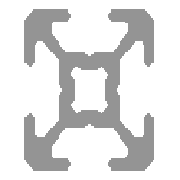
# Autodesk Inventor part: 2020x50mm
Saved by Autodesk Inventor 2015 (Build 190159000, 159)
## iProperties
Created: 2011-02-10
Part Number: 2020x50mm
Document SubType Name: Modeling
Designer: S. Wile
Density: 2.71 g/cm^3
Categories: <MemberInstance><Categories><Category DisplayName="Structural Shapes" InternalName="089c4875-fa83-4c05-b084-43b9cc11f5ed" Mnemonic="GRDR"><CategoryParameter DisplayName="Custom Base Point" InternalName="4f1d1b73-316d-484b-a3df-9cbabb16eb77" Mnemonic="shpBasePoint"/><CategoryParameter DisplayName="FG Authored" InternalName="9c666724-f362-4ea7-ac62-f6a007de5c69" Mnemonic="shpFGAuto"/><CategoryParameter DisplayName="Legacy Member ID" InternalName="340afe4f-75d7-48d3-ab7d-943f3c3da468" Mnemonic="LegacyMemberID"/><CategoryParameter DisplayName="Base Length" InternalName="42e34263-8f20-4d0e-ad48-bf1385b87c24" Mnemonic="shplen"/><CategoryParameter DisplayName="Distance of the Center of Gravity X-X" InternalName="26c9bdb8-9c79-4b4f-a92e-8e197583c9c4" Mnemonic="grcendistX"/><CategoryParameter DisplayName="Distance of the Center of Gravity Y-Y" InternalName="bcc4fb17-7af4-436a-8f8c-d0aa3b0248c5" Mnemonic="grcendistY"/><CategoryParameter DisplayName="Torsional Rigidity Modulus" InternalName="26c1ec35-5026-4c63-ad0a-751cf684a536" Mnemonic="torrigmod"/><CategoryParameter DisplayName="Torsional Section Modulus" InternalName="7c55a8dc-8844-49f9-a867-cc677b30ec9a" Mnemonic="torsecmod"/><CategoryParameter DisplayName="Coefficient of Shear Displacement" InternalName="de4c90c6-aaa8-468f-a335-6737b311b5d3" Mnemonic="shdispc"/><CategoryParameter DisplayName="Section Area" InternalName="1ff91680-64b0-4202-b9a3-7fd3f94bba3b" Mnemonic="secarea"/><CategoryParameter DisplayName="Moment of Inertia (x)" InternalName="4cd780bc-73d7-43ac-917a-579e5cbd684d" Mnemonic="inermomx"/><CategoryParameter DisplayName="Moment of Inertia (y)" InternalName="4b9f58ea-bced-460e-81ea-3d29ca5a49e3" Mnemonic="inermomy"/><CategoryParameter DisplayName="Section Module (x)" InternalName="72cfad18-cf51-4ed4-aaa7-c6b224f8419f" Mnemonic="secmodx"/><CategoryParameter DisplayName="Section Module (y)" InternalName="59eaa5e9-d227-48dc-b6c1-6920f96e0f95" Mnemonic="secmody"/><CategoryParameter DisplayName="Radius of Gyration (x)" InternalName="25778675-03e9-40c1-b6a8-4a9ed693320d" Mnemonic="gyrradx"/><CategoryParameter DisplayName="Radius of Gyration (y)" InternalName="bfa18ebe-1636-4dbe-8d42-b263e0b73184" Mnemonic="gyrrady"/><CategoryParameter DisplayName="Shape Thickness" InternalName="d109cf76-8eb4-42fc-9800-4409734adc67" Mnemonic="shpthick"/><CategoryParameter DisplayName="Second Shape Thickness" InternalName="9251a8e1-85fd-4e47-af99-afdb762317d9" Mnemonic="shpthick2"/><CategoryParameter DisplayName="Shape Width" InternalName="7c717d54-a18f-4666-b4d4-573cce22c62c" Mnemonic="shpwdth"/><CategoryParameter DisplayName="Shape Height" InternalName="50274e7d-5ac0-4796-92cb-c59e54983c67" Mnemonic="shpheig"/><CategoryParameter DisplayName="Mass per Length Unit" InternalName="0bb95a10-148f-4027-a459-38d7b056702a" Mnemonic="shpmass"/><CategoryParameter DisplayName="Section Designation" InternalName="5a64d034-428d-49c8-ba32-7619764de20f" Mnemonic="shpdes"/><Category DisplayName="Other" InternalName="f02205ff-2390-476f-921c-0b3185f88e84" Mnemonic="OTHSHP"><CategoryParameter DisplayName="Moment of Inertia (x)" InternalName="ec6737bc-264f-43ed-b0bd-f6d410c2718d" Mnemonic="inermomx"/><CategoryParameter DisplayName="Moment of Inertia (y)" InternalName="044c654e-f649-48ac-84cc-650a29ae31ca" Mnemonic="inermomy"/><CategoryParameter DisplayName="Section Module (x)" InternalName="cac70804-9d39-43bb-be17-56ea1f39a6c2" Mnemonic="secmodx"/><CategoryParameter DisplayName="Section Module (y)" InternalName="88b8bff9-a616-4028-93d5-ed4f79680d13" Mnemonic="secmody"/><CategoryParameter DisplayName="Section Area" InternalName="c46ecdf8-b6eb-4db9-8b25-30258930c1e3" Mnemonic="secarea"/><CategoryParameter DisplayName="Radius of Gyration (x)" InternalName="ee72c61e-565e-4fd6-b448-66e1e1abcb7e" Mnemonic="gyrradx"/><CategoryParameter DisplayName="Radius of Gyration (y)" InternalName="743e1dfe-1bba-408b-b985-cf752b207386" Mnemonic="gyrrady"/><CategoryParameter DisplayName="Shape Thickness" InternalName="12b1a788-9233-48fd-a933-2df8ff42b15f" Mnemonic="shpthick"/><CategoryParameter DisplayName="Mass per Length Unit" InternalName="2fd289d6-9394-4d2d-97e6-6659d7d4551d" Mnemonic="shpmass"/></Category></Category></Categories><FamilyTemplate Id="20x20"><FamilyTemplateParameters><FamilyTemplateParameter ObjectType="kUserParameterObject" ValueType="xs:double" Id="1" ObjectReferenceKey="Length"/><FamilyTemplateParameter ObjectType="kPropertyObject" ValueType="xs:string" Id="4" ObjectReferenceKey="{32853F0F-3444-11d1-9E93-0060B03C1CA6}" SubObjectId="52"/><FamilyTemplateParameter ObjectType="kPartComponentDefinitionObject" ValueType="xs:string" Id="5" SubObjectId="Material"/><FamilyTemplateParameter ObjectType="kPropertyObject" ValueType="xs:string" Id="6" ObjectReferenceKey="{32853F0F-3444-11d1-9E93-0060B03C1CA6}" SubObjectId="5"/><FamilyTemplateParameter ObjectType="kPropertyObject" ValueType="xs:string" Id="7" ObjectReferenceKey="{32853F0F-3444-11D1-9E93-0060B03C1CA6}" SubObjectId="55"/><FamilyTemplateParameter ObjectType="kiPartTableColumnObject" ValueType="xs:string" Id="18" ObjectReferenceKey="FILENAME"/><FamilyTemplateParameter ObjectType="kiPartTableColumnObject" ValueType="xs:string" Id="19" ObjectReferenceKey="MEMBER_REVISION"/></FamilyTemplateParameters></FamilyTemplate><CategoryParameterMap><ParamToTemplateMap><ParamToTemplate CategoryParameter="//CategoryParameter[@InternalName='9c666724-f362-4ea7-ac62-f6a007de5c69']" ConstantValue="1"/><ParamToTemplate CategoryParameter="//CategoryParameter[@InternalName='2675968c-4ce5-49e0-a4f5-552d29089031']" TemplateParameter="4"/><ParamToTemplate CategoryParameter="//CategoryParameter[@InternalName='8b46a4cc-9585-4fed-90c3-899f57e09a73']" TemplateParameter="18"/><ParamToTemplate CategoryParameter="//CategoryParameter[@InternalName='42e34263-8f20-4d0e-ad48-bf1385b87c24']" TemplateParameter="1"/><ParamToTemplate CategoryParameter="//CategoryParameter[@InternalName='818a152a-d3c3-49ca-80ee-df7d91421b8e']" TemplateParameter="5"/><ParamToTemplate CategoryParameter="//CategoryParameter[@InternalName='a65d44b9-392f-4f4f-857b-e4b3d54996fe']" TemplateParameter="19"/><ParamToTemplate CategoryParameter="//CategoryParameter[@InternalName='016b6077-bfbe-49bd-92c9-d8d59c39c941']" TemplateParameter="6"/></ParamToTemplateMap></CategoryParameterMap></MemberInstance>
Stock Number: 3 842 992 888
Description: PROFILE 20x20, -/-
Material: Aluminum-6061
Mass: 11.2397 g
Surface Area: 47.9691 cm^2
Volume: 4.14751 cm^3
Appearance: Aluminum - Flat-1
RuleStatus: InUse
Author: S. Wile
Autodesk Inventor part; units mm, degrees
ref_plane "YZ Plane" through (0, 0, 0) normal (1, 0, 0) x (0, 1, 0)
ref_plane "XZ Plane" through (0, 0, 0) normal (0, 1, 0) x (-1, 0, 0)
ref_plane "XY Plane" through (0, 0, 0) normal (0, 0, 1) x (1, 0, 0)
sketch "20x20" plane through (0, 0, 0) normal (0, 0, 1) x (1, 0, 0)
  line L0 (-14.2327, 14.1046) -> (-14.2327, 14.8364)
  arc A0 (-14.2327, 14.1046) -> (-13.7327, 13.6046) centre (-13.7327, 14.1046) ccw
  line L1 (-11.7327, 13.6046) -> (-13.7327, 13.6046)
  arc A1 (-11.2327, 13.1046) -> (-11.7327, 13.6046) centre (-11.7327, 13.1046) ccw
  line L2 (-11.2327, 12.8046) -> (-11.2327, 13.1046)
  arc A2 (-11.4327, 12.6046) -> (-11.2327, 12.8046) centre (-11.4327, 12.8046) ccw
  line L3 (-11.5818, 12.6046) -> (-11.4327, 12.6046)
  arc A3 (-11.5818, 12.6046) -> (-11.7818, 12.4046) centre (-11.5818, 12.4046) ccw
  line L4 (-11.7818, 12.3042) -> (-11.7818, 12.4046)
  arc A4 (-11.9818, 12.1042) -> (-11.7818, 12.3042) centre (-11.9818, 12.3042) ccw
  line L5 (-16.7331, 12.1042) -> (-11.9818, 12.1042)
  arc A5 (-18.2331, 13.6042) -> (-16.7331, 12.1042) centre (-16.7331, 13.6042) ccw
  line L6 (-18.2331, 18.3542) -> (-18.2331, 13.6042)
  arc A6 (-18.0331, 18.5542) -> (-18.2331, 18.3542) centre (-18.0331, 18.3542) ccw
  line L7 (-17.9323, 18.5542) -> (-18.0331, 18.5542)
  arc A7 (-17.9323, 18.5542) -> (-17.7323, 18.7542) centre (-17.9323, 18.7542) ccw
  line L8 (-17.7323, 18.9046) -> (-17.7323, 18.7542)
  arc A8 (-17.5323, 19.1046) -> (-17.7323, 18.9046) centre (-17.5323, 18.9046) ccw
  line L9 (-17.2323, 19.1046) -> (-17.5323, 19.1046)
  arc A9 (-16.7323, 18.6046) -> (-17.2323, 19.1046) centre (-17.2323, 18.6046) ccw
  line L10 (-16.7323, 16.6045) -> (-16.7323, 18.6046)
  arc A10 (-16.7323, 16.6045) -> (-16.2323, 16.1045) centre (-16.2323, 16.6045) ccw
  line L11 (-15.5001, 16.1045) -> (-16.2323, 16.1045)
  arc A11 (-15.5001, 16.1045) -> (-15.1465, 16.251) centre (-15.5001, 16.6045) ccw
  line L12 (-12.8787, 18.5188) -> (-15.1465, 16.251)
  arc A12 (-12.8787, 18.5188) -> (-12.7323, 18.8723) centre (-13.2323, 18.8723) ccw
  line L13 (-12.7323, 21.1509) -> (-12.7323, 18.8723)
  arc A13 (-12.7055, 21.2509) -> (-12.7323, 21.1509) centre (-12.5323, 21.1509) ccw
  line L14 (-12.2704, 22.0045) -> (-12.7055, 21.2509)
  arc A14 (-12.2704, 22.0045) -> (-12.2704, 22.2045) centre (-12.4436, 22.1045) ccw
  line L15 (-12.7055, 22.9581) -> (-12.2704, 22.2045)
  arc A15 (-12.7323, 23.0581) -> (-12.7055, 22.9581) centre (-12.5323, 23.0581) ccw
  line L16 (-12.7323, 25.3364) -> (-12.7323, 23.0581)
  arc A16 (-12.7323, 25.3364) -> (-12.8787, 25.69) centre (-13.2323, 25.3364) ccw
  line L17 (-15.1465, 27.9577) -> (-12.8787, 25.69)
  arc A17 (-15.1465, 27.9577) -> (-15.5001, 28.1042) centre (-15.5001, 27.6042) ccw
  line L18 (-16.2323, 28.1042) -> (-15.5001, 28.1042)
  arc A18 (-16.2323, 28.1042) -> (-16.7323, 27.6042) centre (-16.2323, 27.6042) ccw
  line L19 (-16.7323, 25.6038) -> (-16.7323, 27.6042)
  arc A19 (-17.2323, 25.1038) -> (-16.7323, 25.6038) centre (-17.2323, 25.6038) ccw
  line L20 (-17.5323, 25.1038) -> (-17.2323, 25.1038)
  arc A20 (-17.7323, 25.3038) -> (-17.5323, 25.1038) centre (-17.5323, 25.3038) ccw
  line L21 (-17.7323, 25.452) -> (-17.7323, 25.3038)
  arc A21 (-17.7323, 25.452) -> (-17.9323, 25.652) centre (-17.9323, 25.452) ccw
  line L22 (-18.0331, 25.652) -> (-17.9323, 25.652)
  arc A22 (-18.2331, 25.852) -> (-18.0331, 25.652) centre (-18.0331, 25.852) ccw
  line L23 (-18.2331, 30.602) -> (-18.2331, 25.852)
  arc A23 (-16.7331, 32.102) -> (-18.2331, 30.602) centre (-16.7331, 30.602) ccw
  arc A24 (-11.7818, 31.8042) -> (-11.5818, 31.6042) centre (-11.5818, 31.8042) ccw
  line L24 (-11.4327, 31.6042) -> (-11.5818, 31.6042)
  arc A25 (-11.2327, 31.4042) -> (-11.4327, 31.6042) centre (-11.4327, 31.4042) ccw
  line L25 (-11.2327, 31.1042) -> (-11.2327, 31.4042)
  arc A26 (-11.7327, 30.6042) -> (-11.2327, 31.1042) centre (-11.7327, 31.1042) ccw
  line L26 (-13.7327, 30.6042) -> (-11.7327, 30.6042)
  arc A27 (-13.7327, 30.6042) -> (-14.2327, 30.1042) centre (-13.7327, 30.1042) ccw
  line L27 (-14.2327, 29.3723) -> (-14.2327, 30.1042)
  arc A28 (-14.2327, 29.3723) -> (-14.0862, 29.0188) centre (-13.7327, 29.3723) ccw
  line L28 (-11.8181, 26.7506) -> (-14.0862, 29.0188)
  arc A29 (-11.8181, 26.7506) -> (-11.4646, 26.6042) centre (-11.4646, 27.1042) ccw
  line L29 (-9.1859, 26.6042) -> (-11.4646, 26.6042)
  arc A30 (-9.0859, 26.5774) -> (-9.1859, 26.6042) centre (-9.1859, 26.4042) ccw
  line L30 (-8.3323, 26.1423) -> (-9.0859, 26.5774)
  arc A31 (-8.3323, 26.1423) -> (-8.1323, 26.1423) centre (-8.2323, 26.3155) ccw
  line L31 (-7.3787, 26.5774) -> (-8.1323, 26.1423)
  arc A32 (-7.2787, 26.6042) -> (-7.3787, 26.5774) centre (-7.2787, 26.4042) ccw
  line L32 (-5.0004, 26.6042) -> (-7.2787, 26.6042)
  arc A33 (-5.0004, 26.6042) -> (-4.6469, 26.7506) centre (-5.0004, 27.1042) ccw
  line L33 (-2.3787, 29.0188) -> (-4.6469, 26.7506)
  arc A34 (-2.3787, 29.0188) -> (-2.2323, 29.3723) centre (-2.7323, 29.3723) ccw
  line L34 (-2.2323, 30.1042) -> (-2.2323, 29.3723)
  arc A35 (-2.2323, 30.1042) -> (-2.7323, 30.6042) centre (-2.7323, 30.1042) ccw
  line L35 (-4.7327, 30.6042) -> (-2.7323, 30.6042)
  arc A36 (-5.2327, 31.1042) -> (-4.7327, 30.6042) centre (-4.7327, 31.1042) ccw
  line L36 (-5.2327, 31.4042) -> (-5.2327, 31.1042)
  arc A37 (-5.0327, 31.6042) -> (-5.2327, 31.4042) centre (-5.0327, 31.4042) ccw
  line L37 (-4.884, 31.6042) -> (-5.0327, 31.6042)
  arc A38 (-4.884, 31.6042) -> (-4.684, 31.8042) centre (-4.884, 31.8042) ccw
  line L38 (-4.684, 31.902) -> (-4.684, 31.8042)
  arc A39 (-4.484, 32.102) -> (-4.684, 31.902) centre (-4.484, 31.902) ccw
  line L39 (0.2656, 32.102) -> (-4.484, 32.102)
  arc A40 (1.7656, 30.602) -> (0.2656, 32.102) centre (0.2656, 30.602) ccw
  line L40 (1.7656, 25.852) -> (1.7656, 30.602)
  arc A41 (1.5656, 25.652) -> (1.7656, 25.852) centre (1.5656, 25.852) ccw
  line L41 (1.467, 25.652) -> (1.5656, 25.652)
  arc A42 (1.467, 25.652) -> (1.267, 25.452) centre (1.467, 25.452) ccw
  line L42 (1.267, 25.3038) -> (1.267, 25.452)
  arc A43 (1.067, 25.1038) -> (1.267, 25.3038) centre (1.067, 25.3038) ccw
  line L43 (0.767, 25.1038) -> (1.067, 25.1038)
  arc A44 (0.267, 25.6038) -> (0.767, 25.1038) centre (0.767, 25.6038) ccw
  line L44 (0.267, 27.6042) -> (0.267, 25.6038)
  arc A45 (0.267, 27.6042) -> (-0.233, 28.1042) centre (-0.233, 27.6042) ccw
  line L45 (-0.965, 28.1042) -> (-0.233, 28.1042)
  arc A46 (-0.965, 28.1042) -> (-1.3185, 27.9577) centre (-0.965, 27.6042) ccw
  line L46 (-3.5862, 25.6901) -> (-1.3185, 27.9577)
  arc A47 (-3.5862, 25.6901) -> (-3.7326, 25.3365) centre (-3.2326, 25.3365) ccw
  line L47 (-3.7326, 23.0581) -> (-3.7326, 25.3365)
  arc A48 (-3.7594, 22.9581) -> (-3.7326, 23.0581) centre (-3.9326, 23.0581) ccw
  line L48 (-4.1945, 22.2045) -> (-3.7594, 22.9581)
  arc A49 (-4.1945, 22.2045) -> (-4.1945, 22.0045) centre (-4.0213, 22.1045) ccw
  line L49 (-3.7594, 21.2509) -> (-4.1945, 22.0045)
  arc A50 (-3.7326, 21.1509) -> (-3.7594, 21.2509) centre (-3.9326, 21.1509) ccw
  line L50 (-3.7326, 18.8723) -> (-3.7326, 21.1509)
  arc A51 (-3.7326, 18.8723) -> (-3.5862, 18.5187) centre (-3.2326, 18.8723) ccw
  line L51 (-1.3184, 16.251) -> (-3.5862, 18.5187)
  arc A52 (-1.3184, 16.251) -> (-0.9649, 16.1045) centre (-0.9649, 16.6045) ccw
  line L52 (-0.233, 16.1045) -> (-0.9649, 16.1045)
  arc A53 (-0.233, 16.1045) -> (0.267, 16.6045) centre (-0.233, 16.6045) ccw
  line L53 (0.267, 18.6046) -> (0.267, 16.6045)
  arc A54 (0.767, 19.1046) -> (0.267, 18.6046) centre (0.767, 18.6046) ccw
  line L54 (1.067, 19.1046) -> (0.767, 19.1046)
  arc A55 (1.267, 18.9046) -> (1.067, 19.1046) centre (1.067, 18.9046) ccw
  line L55 (1.267, 18.7542) -> (1.267, 18.9046)
  arc A56 (1.267, 18.7542) -> (1.467, 18.5542) centre (1.467, 18.7542) ccw
  line L56 (1.5656, 18.5542) -> (1.467, 18.5542)
  arc A57 (1.7656, 18.3542) -> (1.5656, 18.5542) centre (1.5656, 18.3542) ccw
  line L57 (1.7656, 13.6042) -> (1.7656, 18.3542)
  arc A58 (0.2656, 12.1042) -> (1.7656, 13.6042) centre (0.2656, 13.6042) ccw
  line L58 (-4.484, 12.1042) -> (0.2656, 12.1042)
  arc A59 (-4.684, 12.3042) -> (-4.484, 12.1042) centre (-4.484, 12.3042) ccw
  line L59 (-4.684, 12.4046) -> (-4.684, 12.3042)
  arc A60 (-4.684, 12.4046) -> (-4.884, 12.6046) centre (-4.884, 12.4046) ccw
  line L60 (-5.0327, 12.6046) -> (-4.884, 12.6046)
  arc A61 (-5.2327, 12.8046) -> (-5.0327, 12.6046) centre (-5.0327, 12.8046) ccw
  line L61 (-5.2327, 13.1046) -> (-5.2327, 12.8046)
  arc A62 (-4.7327, 13.6046) -> (-5.2327, 13.1046) centre (-4.7327, 13.1046) ccw
  line L62 (-2.7323, 13.6046) -> (-4.7327, 13.6046)
  arc A63 (-2.7323, 13.6046) -> (-2.2323, 14.1046) centre (-2.7323, 14.1046) ccw
  line L63 (-2.2323, 14.8364) -> (-2.2323, 14.1046)
  arc A64 (-2.2323, 14.8364) -> (-2.3788, 15.19) centre (-2.7323, 14.8364) ccw
  line L64 (-4.6465, 17.4577) -> (-2.3788, 15.19)
  arc A65 (-4.6465, 17.4577) -> (-5.0001, 17.6042) centre (-5.0001, 17.1042) ccw
  line L65 (-7.2787, 17.6042) -> (-5.0001, 17.6042)
  arc A66 (-7.3787, 17.631) -> (-7.2787, 17.6042) centre (-7.2787, 17.8042) ccw
  line L66 (-8.1323, 18.0661) -> (-7.3787, 17.631)
  arc A67 (-8.1323, 18.0661) -> (-8.3323, 18.0661) centre (-8.2323, 17.8929) ccw
  line L67 (-9.0859, 17.631) -> (-8.3323, 18.0661)
  arc A68 (-9.1859, 17.6042) -> (-9.0859, 17.631) centre (-9.1859, 17.8042) ccw
  line L68 (-11.4649, 17.6042) -> (-9.1859, 17.6042)
  arc A69 (-11.4649, 17.6042) -> (-11.8185, 17.4577) centre (-11.4649, 17.1042) ccw
  line L69 (-14.0862, 15.19) -> (-11.8185, 17.4577)
  arc A70 (-14.0862, 15.19) -> (-14.2327, 14.8364) centre (-13.7327, 14.8364) ccw
  line L70 (-11.2243, 24.0126) -> (-10.6774, 23.3609)
  arc A71 (-10.6774, 23.3609) -> (-10.6774, 20.8453) centre (-8.2329, 22.1031) ccw
  line L71 (-10.6774, 20.8453) -> (-11.2243, 20.1936)
  arc A72 (-11.2243, 20.1936) -> (-10.1463, 19.1142) centre (-8.2329, 22.1031) ccw
  line L72 (-10.1463, 19.1142) -> (-9.4907, 19.6586)
  arc A73 (-9.4907, 19.6586) -> (-6.9751, 19.6586) centre (-8.2329, 22.1031) ccw
  line L73 (-6.9751, 19.6586) -> (-6.3194, 19.1142)
  arc A74 (-6.3194, 19.1142) -> (-5.2414, 20.1936) centre (-8.2329, 22.1031) ccw
  line L74 (-5.2414, 20.1936) -> (-5.7884, 20.8453)
  arc A75 (-5.7884, 20.8453) -> (-5.7884, 23.3609) centre (-8.2329, 22.1031) ccw
  line L75 (-5.7884, 23.3609) -> (-5.2414, 24.0126)
  arc A76 (-5.2414, 24.0126) -> (-6.3195, 25.092) centre (-8.2329, 22.1031) ccw
  line L76 (-6.3195, 25.092) -> (-6.9751, 24.5476)
  arc A77 (-6.9751, 24.5476) -> (-9.4906, 24.5477) centre (-8.2329, 22.1031) ccw
  line L77 (-9.4906, 24.5477) -> (-10.1463, 25.092)
  arc A78 (-10.1463, 25.092) -> (-11.2243, 24.0126) centre (-8.2329, 22.1031) ccw
  line L78 (-11.9818, 32.102) -> (-16.7331, 32.102)
  arc A79 (-11.7818, 31.902) -> (-11.9818, 32.102) centre (-11.9818, 31.902) ccw
  line L79 (-11.7818, 31.8042) -> (-11.7818, 31.902)
sketch "Sketch1" plane through (0, 0, 0) normal (0, 0, 1) x (1, 0, 0)
  line L0 (-5.9998, -7.9985) -> (-5.9998, -7.2667)
  arc A0 (-5.9998, -7.9985) -> (-5.4998, -8.4985) centre (-5.4998, -7.9985) ccw
  line L1 (-3.4998, -8.4985) -> (-5.4998, -8.4985)
  arc A1 (-2.9998, -8.9985) -> (-3.4998, -8.4985) centre (-3.4998, -8.9985) ccw
  line L2 (-2.9998, -9.2985) -> (-2.9998, -8.9985)
  arc A2 (-3.1998, -9.4985) -> (-2.9998, -9.2985) centre (-3.1998, -9.2985) ccw
  line L3 (-3.3489, -9.4985) -> (-3.1998, -9.4985)
  arc A3 (-3.3489, -9.4985) -> (-3.5489, -9.6985) centre (-3.3489, -9.6985) ccw
  line L4 (-3.5489, -9.7989) -> (-3.5489, -9.6985)
  arc A4 (-3.7489, -9.9989) -> (-3.5489, -9.7989) centre (-3.7489, -9.7989) ccw
  line L5 (-8.5002, -9.9989) -> (-3.7489, -9.9989)
  arc A5 (-10.0002, -8.4989) -> (-8.5002, -9.9989) centre (-8.5002, -8.4989) ccw
  line L6 (-10.0002, -3.7489) -> (-10.0002, -8.4989)
  arc A6 (-9.8002, -3.5489) -> (-10.0002, -3.7489) centre (-9.8002, -3.7489) ccw
  line L7 (-9.6994, -3.5489) -> (-9.8002, -3.5489)
  arc A7 (-9.6994, -3.5489) -> (-9.4994, -3.3489) centre (-9.6994, -3.3489) ccw
  line L8 (-9.4994, -3.1985) -> (-9.4994, -3.3489)
  arc A8 (-9.2994, -2.9985) -> (-9.4994, -3.1985) centre (-9.2994, -3.1985) ccw
  line L9 (-8.9994, -2.9985) -> (-9.2994, -2.9985)
  arc A9 (-8.4994, -3.4985) -> (-8.9994, -2.9985) centre (-8.9994, -3.4985) ccw
  line L10 (-8.4994, -5.4986) -> (-8.4994, -3.4985)
  arc A10 (-8.4994, -5.4986) -> (-7.9994, -5.9986) centre (-7.9994, -5.4986) ccw
  line L11 (-7.2672, -5.9986) -> (-7.9994, -5.9986)
  arc A11 (-7.2672, -5.9986) -> (-6.9136, -5.8521) centre (-7.2672, -5.4986) ccw
  line L12 (-4.6458, -3.5844) -> (-6.9136, -5.8521)
  arc A12 (-4.6458, -3.5844) -> (-4.4994, -3.2308) centre (-4.9994, -3.2308) ccw
  line L13 (-4.4994, -0.9522) -> (-4.4994, -3.2308)
  arc A13 (-4.4726, -0.8522) -> (-4.4994, -0.9522) centre (-4.2994, -0.9522) ccw
  line L14 (-4.0375, -0.0986) -> (-4.4726, -0.8522)
  arc A14 (-4.0375, -0.0986) -> (-4.0375, 0.1014) centre (-4.2107, 0.0014) ccw
  line L15 (-4.4726, 0.855) -> (-4.0375, 0.1014)
  arc A15 (-4.4994, 0.955) -> (-4.4726, 0.855) centre (-4.2994, 0.955) ccw
  line L16 (-4.4994, 3.2333) -> (-4.4994, 0.955)
  arc A16 (-4.4994, 3.2333) -> (-4.6458, 3.5869) centre (-4.9994, 3.2333) ccw
  line L17 (-6.9136, 5.8546) -> (-4.6458, 3.5869)
  arc A17 (-6.9136, 5.8546) -> (-7.2672, 6.0011) centre (-7.2672, 5.5011) ccw
  line L18 (-7.9994, 6.0011) -> (-7.2672, 6.0011)
  arc A18 (-7.9994, 6.0011) -> (-8.4994, 5.5011) centre (-7.9994, 5.5011) ccw
  line L19 (-8.4994, 3.5007) -> (-8.4994, 5.5011)
  arc A19 (-8.9994, 3.0007) -> (-8.4994, 3.5007) centre (-8.9994, 3.5007) ccw
  line L20 (-9.2994, 3.0007) -> (-8.9994, 3.0007)
  arc A20 (-9.4994, 3.2007) -> (-9.2994, 3.0007) centre (-9.2994, 3.2007) ccw
  line L21 (-9.4994, 3.3489) -> (-9.4994, 3.2007)
  arc A21 (-9.4994, 3.3489) -> (-9.6994, 3.5489) centre (-9.6994, 3.3489) ccw
  line L22 (-9.8002, 3.5489) -> (-9.6994, 3.5489)
  arc A22 (-10.0002, 3.7489) -> (-9.8002, 3.5489) centre (-9.8002, 3.7489) ccw
  line L23 (-10.0002, 8.4989) -> (-10.0002, 3.7489)
  arc A23 (-8.5002, 9.9989) -> (-10.0002, 8.4989) centre (-8.5002, 8.4989) ccw
  arc A24 (-3.5489, 9.7011) -> (-3.3489, 9.5011) centre (-3.3489, 9.7011) ccw
  line L24 (-3.1998, 9.5011) -> (-3.3489, 9.5011)
  arc A25 (-2.9998, 9.3011) -> (-3.1998, 9.5011) centre (-3.1998, 9.3011) ccw
  line L25 (-2.9998, 9.0011) -> (-2.9998, 9.3011)
  arc A26 (-3.4998, 8.5011) -> (-2.9998, 9.0011) centre (-3.4998, 9.0011) ccw
  line L26 (-5.4998, 8.5011) -> (-3.4998, 8.5011)
  arc A27 (-5.4998, 8.5011) -> (-5.9998, 8.0011) centre (-5.4998, 8.0011) ccw
  line L27 (-5.9998, 7.2692) -> (-5.9998, 8.0011)
  arc A28 (-5.9998, 7.2692) -> (-5.8533, 6.9156) centre (-5.4998, 7.2692) ccw
  line L28 (-3.5852, 4.6475) -> (-5.8533, 6.9156)
  arc A29 (-3.5852, 4.6475) -> (-3.2317, 4.5011) centre (-3.2317, 5.0011) ccw
  line L29 (-0.953, 4.5011) -> (-3.2317, 4.5011)
  arc A30 (-0.853, 4.4743) -> (-0.953, 4.5011) centre (-0.953, 4.3011) ccw
  line L30 (-0.0994, 4.0392) -> (-0.853, 4.4743)
  arc A31 (-0.0994, 4.0392) -> (0.1006, 4.0392) centre (0.0006, 4.2124) ccw
  line L31 (0.8542, 4.4743) -> (0.1006, 4.0392)
  arc A32 (0.9542, 4.5011) -> (0.8542, 4.4743) centre (0.9542, 4.3011) ccw
  line L32 (3.2325, 4.5011) -> (0.9542, 4.5011)
  arc A33 (3.2325, 4.5011) -> (3.586, 4.6475) centre (3.2325, 5.0011) ccw
  line L33 (5.8541, 6.9157) -> (3.586, 4.6475)
  arc A34 (5.8541, 6.9157) -> (6.0006, 7.2692) centre (5.5006, 7.2692) ccw
  line L34 (6.0006, 8.0011) -> (6.0006, 7.2692)
  arc A35 (6.0006, 8.0011) -> (5.5006, 8.5011) centre (5.5006, 8.0011) ccw
  line L35 (3.5002, 8.5011) -> (5.5006, 8.5011)
  arc A36 (3.0002, 9.0011) -> (3.5002, 8.5011) centre (3.5002, 9.0011) ccw
  line L36 (3.0002, 9.3011) -> (3.0002, 9.0011)
  arc A37 (3.2002, 9.5011) -> (3.0002, 9.3011) centre (3.2002, 9.3011) ccw
  line L37 (3.3489, 9.5011) -> (3.2002, 9.5011)
  arc A38 (3.3489, 9.5011) -> (3.5489, 9.7011) centre (3.3489, 9.7011) ccw
  line L38 (3.5489, 9.7989) -> (3.5489, 9.7011)
  arc A39 (3.7489, 9.9989) -> (3.5489, 9.7989) centre (3.7489, 9.7989) ccw
  line L39 (8.4985, 9.9989) -> (3.7489, 9.9989)
  arc A40 (9.9985, 8.4989) -> (8.4985, 9.9989) centre (8.4985, 8.4989) ccw
  line L40 (9.9985, 3.7489) -> (9.9985, 8.4989)
  arc A41 (9.7985, 3.5489) -> (9.9985, 3.7489) centre (9.7985, 3.7489) ccw
  line L41 (9.6999, 3.5489) -> (9.7985, 3.5489)
  arc A42 (9.6999, 3.5489) -> (9.4999, 3.3489) centre (9.6999, 3.3489) ccw
  line L42 (9.4999, 3.2007) -> (9.4999, 3.3489)
  arc A43 (9.2999, 3.0007) -> (9.4999, 3.2007) centre (9.2999, 3.2007) ccw
  line L43 (8.9999, 3.0007) -> (9.2999, 3.0007)
  arc A44 (8.4999, 3.5007) -> (8.9999, 3.0007) centre (8.9999, 3.5007) ccw
  line L44 (8.4999, 5.5011) -> (8.4999, 3.5007)
  arc A45 (8.4999, 5.5011) -> (7.9999, 6.0011) centre (7.9999, 5.5011) ccw
  line L45 (7.2679, 6.0011) -> (7.9999, 6.0011)
  arc A46 (7.2679, 6.0011) -> (6.9144, 5.8546) centre (7.2679, 5.5011) ccw
  line L46 (4.6467, 3.5869) -> (6.9144, 5.8546)
  arc A47 (4.6467, 3.5869) -> (4.5003, 3.2334) centre (5.0003, 3.2334) ccw
  line L47 (4.5003, 0.955) -> (4.5003, 3.2334)
  arc A48 (4.4735, 0.855) -> (4.5003, 0.955) centre (4.3003, 0.955) ccw
  line L48 (4.0384, 0.1014) -> (4.4735, 0.855)
  arc A49 (4.0384, 0.1014) -> (4.0384, -0.0986) centre (4.2116, 0.0014) ccw
  line L49 (4.4735, -0.8522) -> (4.0384, -0.0986)
  arc A50 (4.5003, -0.9522) -> (4.4735, -0.8522) centre (4.3003, -0.9522) ccw
  line L50 (4.5003, -3.2308) -> (4.5003, -0.9522)
  arc A51 (4.5003, -3.2308) -> (4.6467, -3.5844) centre (5.0003, -3.2308) ccw
  line L51 (6.9145, -5.8521) -> (4.6467, -3.5844)
  arc A52 (6.9145, -5.8521) -> (7.268, -5.9986) centre (7.268, -5.4986) ccw
  line L52 (7.9999, -5.9986) -> (7.268, -5.9986)
  arc A53 (7.9999, -5.9986) -> (8.4999, -5.4986) centre (7.9999, -5.4986) ccw
  line L53 (8.4999, -3.4985) -> (8.4999, -5.4986)
  arc A54 (8.9999, -2.9985) -> (8.4999, -3.4985) centre (8.9999, -3.4985) ccw
  line L54 (9.2999, -2.9985) -> (8.9999, -2.9985)
  arc A55 (9.4999, -3.1985) -> (9.2999, -2.9985) centre (9.2999, -3.1985) ccw
  line L55 (9.4999, -3.3489) -> (9.4999, -3.1985)
  arc A56 (9.4999, -3.3489) -> (9.6999, -3.5489) centre (9.6999, -3.3489) ccw
  line L56 (9.7985, -3.5489) -> (9.6999, -3.5489)
  arc A57 (9.9985, -3.7489) -> (9.7985, -3.5489) centre (9.7985, -3.7489) ccw
  line L57 (9.9985, -8.4989) -> (9.9985, -3.7489)
  arc A58 (8.4985, -9.9989) -> (9.9985, -8.4989) centre (8.4985, -8.4989) ccw
  line L58 (3.7489, -9.9989) -> (8.4985, -9.9989)
  arc A59 (3.5489, -9.7989) -> (3.7489, -9.9989) centre (3.7489, -9.7989) ccw
  line L59 (3.5489, -9.6985) -> (3.5489, -9.7989)
  arc A60 (3.5489, -9.6985) -> (3.3489, -9.4985) centre (3.3489, -9.6985) ccw
  line L60 (3.2002, -9.4985) -> (3.3489, -9.4985)
  arc A61 (3.0002, -9.2985) -> (3.2002, -9.4985) centre (3.2002, -9.2985) ccw
  line L61 (3.0002, -8.9985) -> (3.0002, -9.2985)
  arc A62 (3.5002, -8.4985) -> (3.0002, -8.9985) centre (3.5002, -8.9985) ccw
  line L62 (5.5006, -8.4985) -> (3.5002, -8.4985)
  arc A63 (5.5006, -8.4985) -> (6.0006, -7.9985) centre (5.5006, -7.9985) ccw
  line L63 (6.0006, -7.2667) -> (6.0006, -7.9985)
  arc A64 (6.0006, -7.2667) -> (5.8541, -6.9131) centre (5.5006, -7.2667) ccw
  line L64 (3.5864, -4.6454) -> (5.8541, -6.9131)
  arc A65 (3.5864, -4.6454) -> (3.2328, -4.4989) centre (3.2328, -4.9989) ccw
  line L65 (0.9542, -4.4989) -> (3.2328, -4.4989)
  arc A66 (0.8542, -4.4721) -> (0.9542, -4.4989) centre (0.9542, -4.2989) ccw
  line L66 (0.1006, -4.037) -> (0.8542, -4.4721)
  arc A67 (0.1006, -4.037) -> (-0.0994, -4.037) centre (0.0006, -4.2102) ccw
  line L67 (-0.853, -4.4721) -> (-0.0994, -4.037)
  arc A68 (-0.953, -4.4989) -> (-0.853, -4.4721) centre (-0.953, -4.2989) ccw
  line L68 (-3.232, -4.4989) -> (-0.953, -4.4989)
  arc A69 (-3.232, -4.4989) -> (-3.5856, -4.6454) centre (-3.232, -4.9989) ccw
  line L69 (-5.8533, -6.9131) -> (-3.5856, -4.6454)
  arc A70 (-5.8533, -6.9131) -> (-5.9998, -7.2667) centre (-5.4998, -7.2667) ccw
  line L70 (-2.9914, 1.9095) -> (-2.4445, 1.2578)
  arc A71 (-2.4445, 1.2578) -> (-2.4445, -1.2578) centre (0, 0) ccw
  line L71 (-2.4445, -1.2578) -> (-2.9914, -1.9095)
  arc A72 (-2.9914, -1.9095) -> (-1.9134, -2.9889) centre (0, 0) ccw
  line L72 (-1.9134, -2.9889) -> (-1.2578, -2.4445)
  arc A73 (-1.2578, -2.4445) -> (1.2578, -2.4445) centre (0, 0) ccw
  line L73 (1.2578, -2.4445) -> (1.9135, -2.9889)
  arc A74 (1.9135, -2.9889) -> (2.9914, -1.9095) centre (0, 0) ccw
  line L74 (2.9914, -1.9095) -> (2.4445, -1.2578)
  arc A75 (2.4445, -1.2578) -> (2.4445, 1.2578) centre (0, 0) ccw
  line L75 (2.4445, 1.2578) -> (2.9914, 1.9095)
  arc A76 (2.9914, 1.9095) -> (1.9134, 2.9889) centre (0, 0) ccw
  line L76 (1.9134, 2.9889) -> (1.2578, 2.4445)
  arc A77 (1.2578, 2.4445) -> (-1.2577, 2.4446) centre (0, 0) ccw
  line L77 (-1.2577, 2.4446) -> (-1.9134, 2.9889)
  arc A78 (-1.9134, 2.9889) -> (-2.9914, 1.9095) centre (0, 0) ccw
  line L78 (-3.7489, 9.9989) -> (-8.5002, 9.9989)
  arc A79 (-3.5489, 9.7989) -> (-3.7489, 9.9989) centre (-3.7489, 9.7989) ccw
  line L79 (-3.5489, 9.7011) -> (-3.5489, 9.7989)
  point P0 (0, 0)
  constraints: 1 other
extrude "Extrusion3" add sketch "Sketch1" along normal blind 50
body "Solid2"
